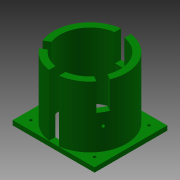
# Autodesk Inventor part: 知能ロボコン外筒改1.1
Saved by Autodesk Inventor 2013 (Build 170138000, 138)
## iProperties
Created: 2014-05-28
Part Number: 知能ロボコン外筒改1.1
Material: ABS プラスチック
Document SubType Name: Modeling
Designer: horumo136
Density: 1 g/cm^3
Author: horumo136
Autodesk Inventor part; units mm, degrees
sketch "スケッチ1" plane through (0, 0, 0) normal (0, 0, 1) x (1, 0, 0)
  circle A0 centre (0, 0) radius 13
  line L0 (0, 13) -> (0, 33)
  circle A1 centre (0, 0) radius 33
  circle A2 centre (0, 0) radius 40
  dimension "d0" = 26
  dimension "d2" = 20
  dimension "d3" = 80
  constraints: 3 coincident, 2 end point, 2 vertical alignment, 1 centre point, 1 vertical, 4 other
  measures "d2" distance of L0.start L0.end
  measures "d3" diameter of A2
extrude "押し出し1" add sketch "スケッチ1" along normal blind 145 contours A2
sketch "スケッチ2" plane through (0, 0, 0) normal (0, 0, -1) x (-1, 0, 0)
  circle A0 centre (0, 0) radius 33 projected
  circle A1 centre (0, 0) radius 40 projected
  line L0 (5.4, 32.5552) -> (-5.4, 32.5552)
  line L1 (0, 0) -> (-10.5703, 0)
  arc A2 (5.4, 32.5552) -> (-5.4, 32.5552) centre (0, 0) ccw
  line L2 (-5.4, 32.5552) -> (5.4, 32.5552)
  line L3 (5.4, 32.5552) -> (5.4, 32.5552)
  line L4 (5.4, 32.5552) -> (-5.4, 32.5552)
  line L5 (-5.4, 32.5552) -> (-5.4, 32.5552)
  line L6 (-5.4, 32.5552) -> (5.4, 32.5552)
  line L7 (5.4, 32.5552) -> (5.4, 33)
  line L8 (5.4, 33) -> (-5.4, 33)
  line L9 (-5.4, 33) -> (-5.4, 32.5552)
  line L10 (-30.8936, -11.6011) -> (-25.4936, -20.9541)
  line L11 (-30.8936, -11.6011) -> (-31.2788, -11.8235)
  line L12 (-31.2788, -11.8235) -> (-25.8788, -21.1765)
  line L13 (-25.8788, -21.1765) -> (-25.4936, -20.9541)
  line L14 (25.4936, -20.9541) -> (30.8936, -11.6011)
  line L15 (25.4936, -20.9541) -> (25.8788, -21.1765)
  line L16 (25.8788, -21.1765) -> (31.2788, -11.8235)
  line L17 (31.2788, -11.8235) -> (30.8936, -11.6011)
  line L18 (-30.8936, -11.6011) -> (-31.2788, -11.8235)
  line L19 (-31.2788, -11.8235) -> (-25.8788, -21.1765)
  line L20 (-25.8788, -21.1765) -> (-25.4936, -20.9541)
  line L21 (-25.4936, -20.9541) -> (-30.8936, -11.6011)
  line L22 (25.4936, -20.9541) -> (25.8788, -21.1765)
  line L23 (25.8788, -21.1765) -> (31.2788, -11.8235)
  line L24 (31.2788, -11.8235) -> (30.8936, -11.6011)
  line L25 (30.8936, -11.6011) -> (25.4936, -20.9541)
  dimension "d6" = 10.8
  dimension "d8" = 10.8
  dimension "d13" = 360
  constraints: 52 end point, 8 parallel, 6 perpendicular, 5 point on circle, 3 horizontal, 1 centre point, 1 collinear, 1 concentric, 31 other
  measures "d6" distance of L0.start L0.end
  measures "d8" distance of L4.end L3.end
extrude "押し出し2" cut sketch "スケッチ2" against normal blind 145 contours L0 A0 | A0 L8 L7 | L17 L16 A0 | A0 L14 | A0 L9 L8 | L16 L15 A0 | L10 A0 | A0 L12 L11 | L13 L12 A0
sketch "スケッチ3" plane through (-5.4, 33, 0) normal (0, -1, 0) x (1, 0, 0)
  line L0 (10.8, 0) -> (10.8, 145) projected
  line L1 (5.4, 0) -> (5.4, 19.5)
  line L2 (5.4, 19.5) -> (5.4, 24.2)
  line L3 (5.4, 24.2) -> (5.4, 74.8)
  circle A0 centre (5.4, 24.2) radius 1.5
  circle A1 centre (5.4, 74.8) radius 1.5
  line L4 (5.4, 74.8) -> (5.4, 79.9)
  line L5 (5.4, 79.9) -> (5.4, 84.6)
  circle A2 centre (5.4, 84.6) radius 1.5
  line L6 (5.4, 84.6) -> (5.4, 135.2)
  circle A3 centre (5.4, 135.2) radius 1.5
  dimension "d15" = 19.5
  dimension "d16" = 4.7
  dimension "d17" = 50.6
  dimension "d18" = 3
  dimension "d19" = 3
  dimension "d20" = 5.1
  dimension "d21" = 4.7
  dimension "d22" = 3
  dimension "d23" = 50.6
  dimension "d24" = 3
  constraints: 12 end point, 5 collinear, 4 centre point, 4 coincident, 1 parallel
  measures "d15" distance of L1.start L1.end
  measures "d16" distance of L1.end L2.end
  measures "d17" distance of L2.end L3.end
  measures "d18" diameter of A0
  measures "d19" diameter of A1
  measures "d20" distance of L4.start L4.end
  measures "d21" distance of L4.end L5.end
  measures "d22" diameter of A2
  measures "d23" distance of L6.start L6.end
  measures "d24" diameter of A3
hole "穴1" at (0, 33, 24.2) at (0, 33, 74.8) at (0, 33, 84.6) at (0, 33, 135.2) direction (0, 1, 0) diameter 3 depth 8 tip angle 118
pattern_circular "円形状パターン1" count 3 over 360 about axis through (0, 0, 0) along (0, 0, 1) of "穴1"
ref_plane "作業平面21" through (-34.641, 20, 0) normal (-0.8660254, 0.5, 0) x (-0.5, -0.8660254, 0)
ref_plane "作業平面18" through (0, 40, 0) normal (0, 1, 0) x (-1, 0, 0)
sketch "スケッチ6" plane through (0, 40, 0) normal (0, 1, 0) x (-1, 0, 0)
  line L0 (0, 0) -> (0, 24.2)
  line L1 (0, 24.2) -> (0, 74.8)
  line L2 (0, 74.8) -> (0, 84.6)
  line L3 (0, 84.6) -> (0, 135.2)
  dimension "d57" = 24.2
  dimension "d58" = 50.6
  dimension "d59" = 9.8
  dimension "d60" = 50.6
  constraints: 8 end point, 4 coincident, 3 collinear, 1 vertical
  measures "d57" distance of L0.start L0.end
  measures "d58" distance of L0.end L1.end
  measures "d59" distance of L1.end L2.end
  measures "d60" distance of L2.end L3.end
hole "穴2" at (0, 40, 74.8) at (0, 40, 24.2) at (0, 40, 84.6) at (0, 40, 135.2) direction (0, -1, 0) diameter 3 depth 8 tip angle 118 counterbore diameter 4 counterbore depth 2
ref_plane "作業平面17" through (0, -40, 0) normal (0, -1, 0) x (1, 0, 0)
sketch "スケッチ7" plane through (0, -40, 0) normal (0, -1, 0) x (1, 0, 0)
  line L0 (0, 0) -> (-5.5, 0)
  line L1 (-5.5, 0) -> (5.5, 0)
  line L2 (-5.5, 0) -> (5.5, 0)
  line L3 (5.5, 0) -> (5.5, 145)
  line L4 (5.5, 145) -> (-5.5, 145)
  line L5 (-5.5, 145) -> (-5.5, 0)
  line L6 (-5.5, 145) -> (5.5, 145)
  line L7 (5.5, 145) -> (5.5, 10)
  line L8 (5.5, 10) -> (-5.5, 10)
  line L9 (-5.5, 10) -> (-5.5, 145)
  dimension "d71" = 5.5
  dimension "d72" = 11
  dimension "d73" = 11
  dimension "d74" = 145
  dimension "d75" = 10
  constraints: 20 end point, 4 parallel, 3 horizontal, 2 perpendicular, 1 collinear, 1 point on line
  measures "d71" distance of L0.start L0.end
  measures "d72" distance of L0.end L1.end
  measures "d73" distance of L4.end L3.end
  measures "d74" distance of L3.end L2.end
  measures "d75" distance between parallel lines of L2 L8
extrude "押し出し4" cut sketch "スケッチ7" against normal blind 10 contours L5 L4 L3 L8
sketch "スケッチ8" plane through (0, 0, 0) normal (0, 0, -1) x (-1, 0, 0)
  circle A0 centre (0, 0) radius 40 projected
  line L0 (5.4, 33) -> (5.4, 32.5552) projected
  line L1 (-5.4, 39.6338) -> (5.4, 39.6338)
  arc A1 (5.4, 39.6338) -> (-5.4, 39.6338) centre (0, 0) ccw
  constraints: 4 point on circle, 2 end point, 1 centre point, 1 concentric, 1 perpendicular
extrude "押し出し5" cut sketch "スケッチ8" against normal blind 145 contours L1 A0 picked at (-0.6016, 39.7423)
sketch "スケッチ9" plane through (0, 0, 0) normal (0, 0, -1) x (-1, 0, 0)
  line L0 (30.8936, -11.6011) -> (31.2788, -11.8235) projected
  line L1 (31.2788, -11.8235) -> (25.8788, -21.1765) projected
  line L2 (25.8788, -21.1765) -> (25.4936, -20.9541) projected
  arc A0 (-25.4936, -20.9541) -> (25.4936, -20.9541) centre (0, 0) ccw projected
  line L3 (-25.4936, -20.9541) -> (-25.8788, -21.1765) projected
  line L4 (-25.8788, -21.1765) -> (-31.2788, -11.8235) projected
  line L5 (-31.2788, -11.8235) -> (-30.8936, -11.6011) projected
  arc A1 (-5.4, 32.5552) -> (-30.8936, -11.6011) centre (0, 0) ccw projected
  line L6 (-5.4, 32.5552) -> (-5.4, 33) projected
  line L7 (-5.4, 33) -> (5.4, 33) projected
  line L8 (5.4, 33) -> (5.4, 32.5552) projected
  arc A2 (30.8936, -11.6011) -> (5.4, 32.5552) centre (0, 0) ccw projected
  line L9 (-45, -40) -> (45, -40)
  line L10 (45, -40) -> (45, 40)
  line L11 (45, 40) -> (-45, 40)
  line L12 (-45, 40) -> (-45, -40)
  line L13 (-45, -40) -> (45, 40) construction
  line L14 (45, -40) -> (-45, 40) construction
  dimension "d80" = 90
  dimension "d81" = 80
  constraints: 12 end point, 2 midpoint, 2 parallel, 1 horizontal, 1 perpendicular
  measures "d80" distance of L11.end L10.end
  measures "d81" distance of L10.end L9.end
extrude "押し出し6" add sketch "スケッチ9" along normal blind 5
sketch "スケッチ10" plane through (0, 0, 145) normal (0, 0, 1) x (1, 0, 0)
  line L0 (5.4, 39.6338) -> (-5.4, 39.6338) projected
  arc A0 (-5.4, 39.6338) -> (-5.5, -39.6201) centre (0, 0) ccw projected
  line L1 (-5.5, -39.6201) -> (-5.5, -32.5384) projected
  arc A1 (-25.4936, -20.9541) -> (-30.8936, -11.6011) centre (0, 0) ccw projected
  line L2 (-25.4936, -20.9541) -> (-25.8788, -21.1765) projected
  line L3 (-25.8788, -21.1765) -> (-31.2788, -11.8235) projected
  line L4 (-31.2788, -11.8235) -> (-30.8936, -11.6011) projected
  arc A2 (-5.4, 32.5552) -> (-30.8936, -11.6011) centre (0, 0) ccw projected
  line L5 (-5.4, 32.5552) -> (-5.4, 33) projected
  line L6 (-5.4, 33) -> (5.4, 33) projected
  line L7 (5.4, 33) -> (5.4, 32.5552) projected
  arc A3 (30.8936, -11.6011) -> (5.4, 32.5552) centre (0, 0) ccw projected
  line L8 (30.8936, -11.6011) -> (31.2788, -11.8235) projected
  line L9 (31.2788, -11.8235) -> (25.8788, -21.1765) projected
  line L10 (25.8788, -21.1765) -> (25.4936, -20.9541) projected
  arc A4 (-5.4, 32.5552) -> (25.4936, -20.9541) centre (0, 0) ccw projected
  line L11 (5.5, -32.5384) -> (5.5, -39.6201) projected
  arc A5 (5.5, -39.6201) -> (5.4, 39.6338) centre (0, 0) ccw projected
  line L12 (-45, 40) -> (45, 40)
  line L13 (45, 40) -> (45, -40)
  line L14 (45, -40) -> (-45, -40)
  line L15 (-45, -40) -> (-45, 40)
  line L16 (-45, 40) -> (45, -40) construction
  line L17 (45, 40) -> (-45, -40) construction
  line L18 (-5.5, -32.5384) -> (-5.5, -40)
  line L19 (-5.5, -40) -> (-45, -40)
  line L20 (-45, -40) -> (-45, 40)
  line L21 (-45, 40) -> (45, 40)
  line L22 (45, 40) -> (45, -40)
  line L23 (45, -40) -> (5.5, -40)
  line L24 (5.5, -40) -> (5.5, -32.5384)
  arc A6 (5.5, -32.5384) -> (-5.5, -32.5384) centre (0, 0) ccw
  circle A7 centre (0, 0) radius 33
  line L25 (-5.5, -40) -> (5.5, -40)
  dimension "d84" = 90
  dimension "d85" = 80
  constraints: 28 end point, 4 collinear, 3 parallel, 2 concentric, 2 midpoint, 2 perpendicular, 2 point on circle, 2 point on line, 1 centre point, 1 coincident, 1 horizontal, 3 other
  measures "d84" distance of L13.end L14.end
  measures "d85" distance of L12.end L13.end
extrude "押し出し7" add sketch "スケッチ10" along normal blind 5 contours A5 L11 A1 L10 L9 L8 L7 L6 L5 L4 L3 L2 L1 A0 L0 | L0 A0 L18 L14 L15 L12 L13 L24 A5 | L24 L14 L18 L1 A1 L11
ref_plane "作業平面16" through (0, 40, 72.5) normal (0, 0, 1) x (1, 0, 0)
sketch "スケッチ12" plane through (0, 40, 72.5) normal (0, 0, 1) x (1, 0, 0)
  line L0 (-45, 0) -> (45, 0)
  line L1 (45, 0) -> (45, -80)
  line L2 (45, -80) -> (-45, -80)
  line L3 (-45, -80) -> (-45, 0)
  line L4 (-45, 0) -> (45, -80) construction
  line L5 (45, 0) -> (-45, -80) construction
  point P0 (0, -40)
  dimension "d90" = 90
  dimension "d91" = 80
  constraints: 12 end point, 2 midpoint, 2 parallel, 1 horizontal, 1 perpendicular
  measures "d90" distance of L1.end L2.end
  measures "d91" distance of L0.end L1.end
extrude "押し出し8" cut sketch "スケッチ12" along normal blind 80
sketch "スケッチ13" plane through (0, 40, 72.5) normal (0, 0, 1) x (1, 0, 0)
  line L0 (25.8788, -61.1765) -> (31.2788, -51.8235) projected
  line L1 (25.4936, -60.9541) -> (25.8788, -61.1765) projected
  arc A0 (-5.4, -7.4448) -> (25.4936, -60.9541) centre (0, -40) ccw projected
  line L2 (5.5, -79.6201) -> (5.5, -72.5384) projected
  arc A1 (-36.4674, -23.5644) -> (5.4, -0.3662) centre (0, -40) ccw projected
  line L3 (-5.4, -0.3662) -> (5.4, -0.3662) projected
  arc A2 (-5.4, -0.3662) -> (5.4, -0.3662) centre (0, -40) ccw projected
  line L4 (-5.5, -72.5384) -> (-5.5, -79.6201) projected
  arc A3 (-25.4936, -60.9541) -> (-26.3681, -20.1576) centre (0, -40) ccw projected
  line L5 (-25.8788, -61.1765) -> (-25.4936, -60.9541) projected
  line L6 (-31.2788, -51.8235) -> (-25.8788, -61.1765) projected
  line L7 (-30.8936, -51.6011) -> (-31.2788, -51.8235) projected
  arc A4 (-5.4, -7.4448) -> (-30.8936, -51.6011) centre (0, -40) ccw projected
  line L8 (-5.4, -7) -> (-5.4, -7.4448) projected
  line L9 (5.4, -7) -> (-5.4, -7) projected
  line L10 (5.4, -7.4448) -> (5.4, -7) projected
  arc A5 (30.8936, -51.6011) -> (5.4, -7.4448) centre (0, -40) ccw projected
  line L11 (31.2788, -51.8235) -> (30.8936, -51.6011) projected
extrude "押し出し9" cut sketch "スケッチ13" against normal blind 5 contours L0 L11 A3 L10 L9 L8 A0 L7 L6 L5 L4 A1 A2 L3 L2 L1
sketch "スケッチ14" plane through (-5.4, 33, -5) normal (0, -1, 0) x (1, 0, 0)
  line L0 (10.8, 0) -> (10.8, 155) projected
  line L1 (0, 72.5) -> (10.8, 72.5)
  line L2 (10.8, 72.5) -> (10.8, 42.5)
  line L3 (10.8, 42.5) -> (0, 42.5)
  line L4 (0, 42.5) -> (0, 72.5)
  point P0 (5.4, 5)
  dimension "d96" = 30
  constraints: 8 end point, 2 parallel, 1 horizontal, 1 perpendicular, 1 point on line
  measures "d96" distance of L1.end L2.end
extrude "押し出し10" cut sketch "スケッチ14" against normal blind 10
sketch "スケッチ15" plane through (31.2788, -11.8235, -5) normal (-0.8660254, 0.5, 0) x (0, 0, 1)
  line L0 (72.5, -10.8) -> (72.5, 0) projected
  line L1 (72.5, 0) -> (0, 0) projected
  line L2 (72.5, -10.8) -> (42.5, -10.8)
  line L3 (42.5, -10.8) -> (42.5, 0)
  line L4 (42.5, 0) -> (72.5, 0)
  line L5 (72.5, 0) -> (72.5, -10.8)
  point P0 (5, -5.4)
  point P1 (155, 0)
  dimension "d100" = 30
  constraints: 8 end point, 2 parallel, 1 horizontal, 1 perpendicular, 1 point on line
  measures "d100" distance of L3.end L4.end
extrude "押し出し11" cut sketch "スケッチ15" against normal blind 10
sketch "スケッチ16" plane through (-25.8788, -21.1765, 67.5) normal (0.8660254, 0.5, 0) x (0, 0, -1)
  line L0 (0, 10.8) -> (0, 0) projected
  line L1 (0, 0) -> (72.5, 0) projected
  line L2 (0, 10.8) -> (30, 10.8)
  line L3 (30, 10.8) -> (30, 0)
  line L4 (30, 0) -> (0, 0)
  line L5 (0, 0) -> (0, 10.8)
  point P0 (67.5, 5.4)
  point P1 (-82.5, 0)
  dimension "d103" = 30
  constraints: 8 end point, 2 parallel, 1 horizontal, 1 perpendicular, 1 point on line
  measures "d103" distance of L3.end L4.end
extrude "押し出し12" cut sketch "スケッチ16" against normal blind 10
sketch "スケッチ17" plane through (0, 0, -5) normal (0, 0, -1) x (-1, 0, 0)
  line L0 (-45, 40) -> (-35, 40)
  line L1 (-35, 40) -> (-35, 30)
  line L2 (-35, 30) -> (-45, 30)
  line L3 (-45, 30) -> (-45, 40)
  line L4 (-45, -40) -> (-35, -40)
  line L5 (-35, -40) -> (-35, -30)
  line L6 (-35, -30) -> (-45, -30)
  line L7 (-45, -30) -> (-45, -40)
  line L8 (45, 40) -> (35, 40)
  line L9 (35, 40) -> (35, 30)
  line L10 (35, 30) -> (45, 30)
  line L11 (45, 30) -> (45, 40)
  line L12 (45, -40) -> (35, -40)
  line L13 (35, -40) -> (35, -30)
  line L14 (35, -30) -> (45, -30)
  line L15 (45, -30) -> (45, -40)
  dimension "d106" = 10
  dimension "d107" = 10
  dimension "d108" = 10
  dimension "d109" = 10
  dimension "d110" = 10
  dimension "d111" = 10
  dimension "d112" = 10
  dimension "d113" = 10
  constraints: 32 end point, 8 parallel, 4 coincident, 4 horizontal, 4 perpendicular
  measures "d106" distance of L1.end L2.end
  measures "d107" distance of L0.end L1.end
  measures "d108" distance of L6.end L5.end
  measures "d109" distance of L5.end L4.end
  measures "d110" distance of L10.end L9.end
  measures "d111" distance of L9.end L8.end
  measures "d112" distance of L13.end L14.end
  measures "d113" distance of L12.end L13.end
hole "穴3" at (35, 30, -5) at (35, -30, -5) at (-35, -30, -5) at (-35, 30, -5) direction (0, 0, 1) diameter 3 depth 10 tip angle 118
sketch "スケッチ18" plane through (0, 0, 10) normal (0, 0, 1) x (1, 0, 0)
  arc A0 (-5.5, -32.5384) -> (5.5, -32.5384) centre (0, 0) ccw projected
  line L0 (-5.5, -39.6201) -> (-5.5, -32.5384) projected
  arc A1 (-5.5, -39.6201) -> (5.5, -39.6201) centre (0, 0) ccw projected
  line L1 (5.5, -39.6201) -> (5.5, -32.5384) projected
extrude "押し出し13" cut sketch "スケッチ18" against normal blind 10
